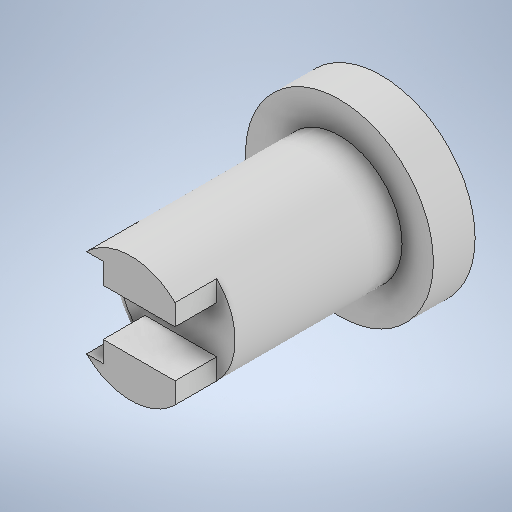
# Autodesk Inventor part: magnet_mount
Saved by Autodesk Inventor 2025.2 (Build 292293000, 293)
## iProperties
Created: 2025-03-10
Part Number: magnet_mount
Material: Generic
Document SubType Name: Modeling
Designer: 3lin2
Density: 1 g/cm^3
Appearance: Default
Author: 3lin2
Autodesk Inventor part; units mm, degrees
ref_plane "YZ Plane" through (0, 0, 0) normal (1, 0, 0) x (0, 1, 0)
ref_plane "XZ Plane" through (0, 0, 0) normal (0, 1, 0) x (-1, 0, 0)
ref_plane "XY Plane" through (0, 0, 0) normal (0, 0, 1) x (1, 0, 0)
sketch "Sketch1" plane through (0, 0, 0) normal (0, 0, 1) x (1, 0, 0)
  circle A0 centre (0, 0) radius 28.575
  dimension "d0" = 57.15
  constraints: 1 centre point, 1 coincident
  measures "d0" diameter of A0
extrude "Extrusion1" add sketch "Sketch1" along normal blind 12.7
sketch "Sketch2" plane through (0, 0, 0) normal (0, 0, -1) x (-1, 0, 0)
  circle A0 centre (0, 0) radius 22.86
  dimension "d3" = 45.72
  constraints: 1 centre point, 1 coincident
  measures "d3" diameter of A0
extrude "Extrusion2" cut sketch "Sketch2" against normal blind 6.35
sketch "Sketch3" plane through (0, 0, 6.35) normal (0, 0, -1) x (-1, 0, 0)
  circle A0 centre (0, 0) radius 10.795
  dimension "d6" = 21.59
  constraints: 1 centre point, 1 coincident
  measures "d6" diameter of A0
extrude "Extrusion3" add sketch "Sketch3" along normal blind 6.35
sketch "Sketch4" plane through (0, 0, 12.7) normal (0, 0, 1) x (1, 0, 0)
  point P0 (0, 0)
sketch "Sketch5" plane through (0, 0, 12.7) normal (0, 0, 1) x (1, 0, 0)
  circle A0 centre (0, 0) radius 19.05
  dimension "d9" = 38.1
  constraints: 1 centre point, 1 coincident
  measures "d9" diameter of A0
extrude "Extrusion4" add sketch "Sketch5" along normal blind 6.35
extrude "Extrusion5" add sketch "Sketch5" along normal blind 50.8
sketch "Sketch6" plane through (0, 0, 63.5) normal (0, 0, 1) x (1, 0, 0)
  circle A0 centre (0, 0) radius 19.05 projected
  arc A1 (13.4629, 13.4778) -> (-13.4629, 13.4778) centre (0, 0) ccw
  line L0 (-13.4629, 13.4778) -> (13.4629, 13.4778)
  arc A2 (-13.4629, -13.4778) -> (13.4629, -13.4778) centre (0, 0) ccw
  line L1 (-13.4629, -13.4778) -> (13.4629, -13.4778)
  constraints: 8 point on circle, 4 end point, 2 centre point, 2 horizontal, 1 concentric
extrude "Extrusion6" add sketch "Sketch6" along normal blind 12.7 contours L0 A0 | A0 L1
fillet "Fillet1" radius 3.175 1 edges at (-19.05, 0, 63.5)
sketch "Sketch7" plane through (-13.4629, 13.4778, 76.2) normal (0, -1, 0) x (1, 0, 0)
  line L0 (0, 0) -> (26.9259, 0) projected
  line L1 (26.9259, -12.7) -> (5.0746, -12.7) projected
  line L2 (26.9259, 0) -> (5.0746, 0)
  line L3 (5.0746, 0) -> (5.0746, -12.7)
  line L4 (5.0746, -12.7) -> (26.9259, -12.7)
  line L5 (26.9259, -12.7) -> (26.9259, 0)
  point P0 (13.4629, -76.2)
  constraints: 8 end point, 2 parallel, 1 horizontal, 1 perpendicular
extrude "Extrusion7" add sketch "Sketch7" along normal blind 6.35
sketch "Sketch8" plane through (-13.4629, -13.4778, 76.2) normal (0, 1, 0) x (1, 0, 0)
  line L0 (5.0746, 12.7) -> (26.9259, 12.7) projected
  line L1 (26.9259, 12.7) -> (26.9259, 0) projected
  line L2 (5.0746, 12.7) -> (26.9259, 12.7)
  line L3 (26.9259, 12.7) -> (26.9259, 0)
  line L4 (26.9259, 0) -> (5.0746, 0)
  line L5 (5.0746, 0) -> (5.0746, 12.7)
  point P0 (13.4629, 76.2)
  constraints: 8 end point, 2 parallel, 1 horizontal, 1 perpendicular
extrude "Extrusion8" add sketch "Sketch8" along normal blind 6.35
body "Solid1"
